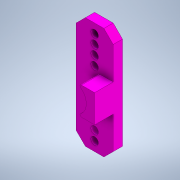
# Autodesk Inventor part: ShaftRest
Saved by Autodesk Inventor 2020 (Build 240168000, 168)
## iProperties
Created: 2020-01-19
Part Number: ShaftRest
Material: Generic
Document SubType Name: Modeling
Designer: srini
Density: 1 g/cm^3
Appearance: Magenta
Author: srini
Autodesk Inventor part; units mm, degrees
ref_plane "YZ Plane" through (0, 0, 0) normal (1, 0, 0) x (0, 1, 0)
ref_plane "XZ Plane" through (0, 0, 0) normal (0, 1, 0) x (-1, 0, 0)
ref_plane "XY Plane" through (0, 0, 0) normal (0, 0, 1) x (1, 0, 0)
sketch "Sketch1" plane through (0, 0, 0) normal (0, 0, 1) x (1, 0, 0)
  line L0 (0, 275.5779) -> (25.4, 275.5779)
  line L1 (25.4, 275.5779) -> (25.4, 351.7779)
  line L2 (25.4, 351.7779) -> (0, 351.7779)
  line L3 (0, 351.7779) -> (0, 275.5779)
  line L4 (0, 0) -> (0, 457.2) projected
  line L5 (25.4, 0) -> (25.4, 457.2) projected
  dimension "d0" = 76.2
  dimension "d1" = 25.4
  constraints: 8 end point, 2 parallel, 1 collinear, 1 horizontal, 1 perpendicular
  measures "d0" distance of L2.end L0.start
  measures "d1" distance of L1.end L2.end
extrude "Extrusion1" add sketch "Sketch1" along normal blind 6.35
sketch "Sketch2" plane through (0, 0, 6.35) normal (0, 0, 1) x (1, 0, 0)
  circle A0 centre (12.7, 281.9279) radius 2.5797
  line L0 (25.4, 275.5779) -> (25.4, 351.7779) projected
  line L1 (0, 275.5779) -> (25.4, 275.5779) projected
  circle A1 centre (12.7, 288.2779) radius 2.5797
  circle A2 centre (12.7, 294.6279) radius 2.5797
  circle A3 centre (12.7, 300.9779) radius 2.5797
  circle A4 centre (12.7, 326.3779) radius 2.5797
  circle A5 centre (12.7, 332.7279) radius 2.5797
  circle A6 centre (12.7, 339.0779) radius 2.5797
  circle A7 centre (12.7, 345.4279) radius 2.5797
  point P0 (0, 0)
  dimension "d4" = 12.7
  dimension "d5" = 6.35
  dimension "d6" = 5.1594
  dimension "d9" = 6.35
  dimension "d16" = 44.45
  constraints: 8 centre point, 2 vertical, 14 other
  measures "d4" distance from line of A0.centre L0
  measures "d5" distance from line of A0.centre L1
  measures "d6" diameter of A0
  measures "d9" distance of A0.centre A1.centre
  measures "d16" distance of A0.centre A4.centre
extrude "Extrusion2" cut sketch "Sketch2" against normal through all
sketch "Sketch3" plane through (0, 0, 6.35) normal (0, 0, 1) x (1, 0, 0)
  line L0 (10.16, 304.1529) -> (25.4, 304.1529)
  line L1 (25.4, 304.1529) -> (25.4, 323.2029)
  line L2 (25.4, 323.2029) -> (10.16, 323.2029)
  line L3 (10.16, 323.2029) -> (10.16, 304.1529)
  line L4 (25.4, 275.5779) -> (25.4, 351.7779) projected
  line L5 (25.4, 351.7779) -> (0, 351.7779) projected
  circle A0 centre (10.16, 313.6779) radius 9.525
  point P0 (0, 0)
  point P1 (10.16, 304.1529)
  point P2 (10.16, 323.2029)
  dimension "d23" = 15.24
  dimension "d24" = 28.575
  dimension "d25" = 19.05
  constraints: 8 end point, 2 parallel, 1 centre point, 1 collinear, 1 horizontal, 1 midpoint, 1 perpendicular, 1 tangent
  measures "d23" distance of L1.end L2.end
  measures "d24" distance between parallel lines of L5 L2
  measures "d25" distance of L2.end L0.start
extrude "Extrusion3" add sketch "Sketch3" along normal blind 12.7 contours A0 L2 L1 L0
fillet "Fillet1" radius 1.016 2 edges at (10.16, 304.1529, 12.7) (10.16, 323.2029, 12.7)
chamfer "Chamfer1" distance 6.35 angle 45 4 edges at (25.4, 351.7779, 3.175) (0, 351.7779, 3.175) (0, 275.5779, 3.175) (25.4, 275.5779, 3.175)
body "Solid1"
